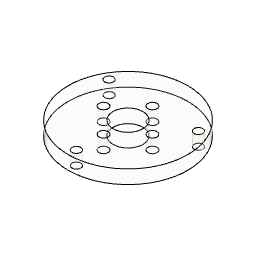
Support_moteur_KOSMOS3-0 (Autodesk Fusion 360 design; units mm, degrees)
Autodesk Fusion 360 part; units mm, degrees
note: some values were not read from the file. Set by a fixed rule: which sketch regions a step uses.
sketch "Esquisse1" plane through (0, 0, 0) normal (0, 0, 1) x (1, 0, 0)
  circle A0 centre (0, 0) radius 22
  circle A1 centre (0, -9) radius 1.7
  circle A2 centre (0, 0) radius 5.5
  circle A3 centre (9, 0) radius 1.7
  circle A4 centre (0, 9) radius 1.7
  circle A5 centre (-9, 0) radius 1.7
  line L0 (0, 0) -> (0, -22) construction
  line L1 (0, 0) -> (0, -20) construction
  line L2 (0, 0) -> (20, 0) construction
  circle A6 centre (0, -19) radius 1.6
  circle A7 centre (16.4545, 9.5) radius 1.6
  circle A8 centre (-16.4545, 9.5) radius 1.6
  point P0 (2.1213, -9.1924)
  point P1 (9.1924, -2.1213)
  point P2 (2.1213, -9.1924)
  point P3 (9.1924, -2.1213)
  point P4 (6.364, -13.435)
  point P5 (13.435, -6.364)
  dimension "d1" = 44
  dimension "d2" = 3.4
  dimension "d3" = 9
  dimension "d4" = 11
  dimension "d6" = 360
  dimension "d17" = 90
  dimension "d18" = 3.2
  dimension "d19" = 19
  dimension "d21" = 360
  constraint coincident A0.centre A2.centre
  constraint coincident A0 L0.end
  constraint vertical L0
  constraint horizontal L2
  constraint coincident L1 A6.centre
  measures "d1" diameter of A0
  measures "d2" diameter of A1
  measures "d3" distance of A0.centre A1.centre
  measures "d4" diameter of A2
  measures "d17" angle of L1 L2
  measures "d18" diameter of A6
  measures "d19" distance of A0.centre A6.centre
extrude "Extrusion1" add sketch "Esquisse1" along normal blind 5
